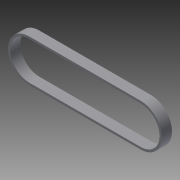
# Autodesk Inventor part: Chassis_7.67inBelt
Saved by Autodesk Inventor 2014 (Build 180170000, 170)
## iProperties
Created: 2016-01-28
Part Number: Chassis_7.67inBelt
Material: Generic
Document SubType Name: Modeling
Designer: choices
Density: 1 g/cm^3
Appearance: Default
Author: choices
Autodesk Inventor part; units mm, degrees
ref_plane "YZ Plane" through (0, 0, 0) normal (1, 0, 0) x (0, 1, 0)
ref_plane "XZ Plane" through (0, 0, 0) normal (0, 1, 0) x (-1, 0, 0)
ref_plane "XY Plane" through (0, 0, 0) normal (0, 0, 1) x (1, 0, 0)
sketch "Sketch1" plane through (0, 0, 0) normal (0, 0, 1) x (1, 0, 0)
  arc A0 (-210.4144, 46.4953) -> (-210.4144, -19.5447) centre (-210.4144, 13.4753) ccw
  arc A1 (-15.5964, -19.5447) -> (-15.5964, 46.4953) centre (-15.5964, 13.4753) ccw
  line L0 (-210.4144, 46.4953) -> (-15.5964, 46.4953)
  line L1 (-210.4144, -19.5447) -> (-15.5964, -19.5447)
  arc A2 (-15.5964, -23.3547) -> (-15.5964, 50.3053) centre (-15.5964, 13.4753) ccw
  line L2 (-15.5964, -23.3547) -> (-210.4144, -23.3547)
  arc A3 (-210.4144, 50.3053) -> (-210.4144, -23.3547) centre (-210.4144, 13.4753) ccw
  line L3 (-210.4144, 50.3053) -> (-15.5964, 50.3053)
  point P0 (0, 0)
  dimension "d0" = 66.04
  dimension "d1" = 66.04
  dimension "d2" = 194.818
  dimension "d3" = 3.81
  constraints: 10 end point, 8 point on circle, 4 centre point, 2 parallel, 2 tangent, 1 horizontal, 3 other
  measures "d0" diameter of A0
  measures "d1" diameter of A1
  measures "d2" distance of A1.centre A0.centre
  measures "d3" distance between parallel lines of L0 L3
extrude "Extrusion1" add sketch "Sketch1" along normal blind 17.78
body "Solid1"
